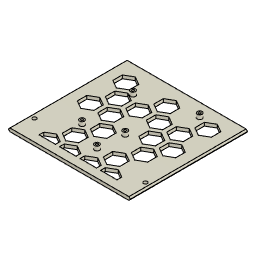
MCU Tray - BTT SKR E3 (Autodesk Fusion 360 design; units mm, degrees)
Autodesk Fusion 360 part; units mm, degrees
note: some values were not read from the file. Chosen so that the rebuilt part matches the saved one: a direction.
imported_body "Derived Base Feature3" makes body 1
imported_body "Derived Base Feature4" makes body 2
imported_body "Derived Base Feature5" makes body 3
imported_body "Derived Base Feature6" makes body 4
sketch "Base" plane through (0, 0, 0) normal (0, 1, 0) x (1, 0, 0)
  line L0 (72.5, 2) -> (-72.5, 2)
  line L1 (-72.5, 2) -> (-72.5, -2) construction
  line L2 (-72.5, -2) -> (72.5, -2)
  line L3 (72.5, -2) -> (72.5, 2) construction
  line L4 (72.5, 2) -> (-72.5, -2) construction
  line L5 (-72.5, 2) -> (72.5, -2) construction
  line L6 (-72.5, 0) -> (-74.3, 0) construction
  line L7 (-72.5, -2) -> (-74.3, -0.2)
  line L8 (-74.3, 0.2) -> (-72.5, 2)
  line L9 (-74.3, -0.2) -> (-74.3, 0)
  line L10 (-74.3, 0) -> (-74.3, 0.2)
  line L11 (0, 0) -> (0, -2) construction
  line L12 (72.5, -2) -> (74.3, -0.2)
  line L13 (74.3, -0.2) -> (74.3, 0)
  line L14 (74.3, 0) -> (74.3, 0.2)
  line L15 (74.3, 0.2) -> (72.5, 2)
  dimension "d1" = 145
  dimension "d2" = 4
  dimension "d3" = 0.2
  constraint horizontal L0
  constraint perpendicular L0 L1
  constraint parallel L0 L2
  constraint parallel L1 L3
  constraint coincident L4 L11.start
  constraint coincident L5 L11.start
  constraint coincident L11.start origin
  constraint midpoint L1 L6.start
  constraint perpendicular L1 L6
  constraint coincident L5 L0.end
  constraint coincident L0 L1.start
  constraint perpendicular L6 L9
  constraint perpendicular L6 L10
  constraint midpoint L2 L11.end
  constraint symmetric L1.end L11 L2.end
  constraint symmetric L0.end L11 L0.start
  constraint symmetric L7.end L11 L12.end
  constraint symmetric L6.end L11 L13.end
  constraint symmetric L8.start L11 L14.end
  measures "d1" distance of L1.end L2.end
  measures "d2" distance of L0.end L1.end
  measures "d3" distance of L7.end L6.end
extrude "Extrude1" add sketch "Base" along normal blind 190 and the other way blind 15 separate body makes body 5
sketch "Tray Mounting Holes" plane through (0, 0, 2) normal (0, 0, 1) x (-1, 0, 0)
  line L0 (72.5, 15) -> (-72.5, 15)
  line L1 (-72.5, 15) -> (-72.5, -190)
  line L2 (-72.5, -190) -> (72.5, -190)
  line L3 (72.5, -190) -> (72.5, 15)
  line L4 (0, 0) -> (0, -13.083) construction
  circle A0 centre (-67.6414, -16.9998) radius 2.3
  line L5 (72.6414, -59.8458) -> (72.6414, 0.0002) construction
  circle A1 centre (67.6414, -16.9998) radius 2.3
  line L6 (72.5, -190) -> (72.5, 15)
  line L7 (72.6414, 0.0002) -> (78.5, 0.0002)
  line L8 (72.6414, 0.0002) -> (67.6414, 0.0002) construction
  line L9 (67.6414, 0.0002) -> (67.6414, -16.9998) construction
  line L10 (67.6414, -16.9998) -> (72.6414, -16.9998) construction
  line L11 (72.6414, -16.9998) -> (72.6414, 0.0002) construction
  dimension "d14" = 5
  dimension "d15" = 17
  dimension "d16" = 4.6
  constraint coincident L4.start origin
  constraint vertical L4
  constraint symmetric L4 A0 A1
  constraint horizontal L8
  constraint vertical L9
  constraint horizontal L10
  constraint vertical L11
  constraint coincident L5.end L7.start
  constraint coincident A1.centre L9.end
  measures "d14" distance of L5.end L8.end
  measures "d15" distance of L5.end L10.end
  measures "d16" diameter of A1
extrude "Extrude2" cut sketch "Tray Mounting Holes" against normal up to surface (4 mm away) contours A0 | A1 bodies 5
extrude "Extrude3" cut 1 faces at (24.1667, 190, 0.6667) along direction (0, -1, 0) blind 40.154 on bodies 5 bodies 5
sketch "MCU Mount Standoffs" plane through (0, 0, 2) normal (0, 0, 1) x (-1, 0, 0)
  line L0 (-72.5, -149.846) -> (72.5, -149.846)
  line L1 (72.5, -149.846) -> (72.5, 15)
  line L2 (72.5, 15) -> (-72.5, 15)
  line L3 (-72.5, 15) -> (-72.5, -149.846)
  circle A0 centre (67.6414, -16.9998) radius 2.3
  circle A1 centre (-67.6414, -16.9998) radius 2.3
  circle A2 centre (-45, 10.1542) radius 3 construction
  circle A3 centre (-45, -139.8458) radius 3 construction
  line L4 (0, -126.2101) -> (0, -149.846) construction
  line L5 (0, -126.2101) -> (0, -22.8658) construction
  line L6 (-32.235, -22.8658) -> (32.235, -22.8658) construction
  line L7 (32.235, -22.8658) -> (32.235, -118.5458) construction
  line L8 (32.235, -118.5458) -> (-32.235, -118.5458) construction
  line L9 (-32.235, -118.5458) -> (-32.235, -22.8658) construction
  circle A4 centre (-32.235, -118.5458) radius 1.4
  circle A5 centre (-32.235, -118.5458) radius 3
  line L10 (32.235, -22.8658) -> (-2.745, -22.8658) construction
  circle A6 centre (-2.745, -22.8658) radius 1.4
  circle A7 centre (-2.745, -22.8658) radius 3
  line L11 (32.235, -22.8658) -> (-5.395, -22.8658) construction
  line L12 (-5.395, -22.8658) -> (-5.395, -54.6658) construction
  circle A8 centre (-5.395, -54.6658) radius 1.4
  circle A9 centre (-5.395, -54.6658) radius 3
  line L13 (32.235, -70.7058) -> (-32.235, -70.7058) construction
  circle A10 centre (32.235, -101.7808) radius 1.4
  circle A11 centre (32.235, -101.7808) radius 3
  circle A12 centre (32.235, -39.6308) radius 1.4
  circle A13 centre (32.235, -39.6308) radius 3
  point P0 (0, -75.2851)
  dimension "d60" = 64.47
  dimension "d61" = 95.68
  dimension "d62" = 2.8
  dimension "d63" = 6
  dimension "d64" = 34.98
  dimension "d65" = 2.8
  dimension "d66" = 6
  dimension "d67" = 37.63
  dimension "d68" = 31.8
  dimension "d69" = 2.8
  dimension "d70" = 6
  dimension "d73" = 2.8
  dimension "d74" = 6
  dimension "d75" = 62.15
  constraint midpoint L0 L4.end
  constraint vertical L4
  constraint vertical L5
  constraint horizontal L6
  constraint perpendicular L6 L7
  constraint parallel L6 L8
  constraint parallel L7 L9
  constraint coincident L8.end L9.start
  constraint coincident L6 L5.end
  constraint coincident L5 P0
  constraint perpendicular L7 L10
  constraint coincident L10.end A6.centre
  constraint perpendicular L7 L11
  constraint perpendicular L6 L12
  constraint coincident L12.end A8.centre
  constraint midpoint L7 L13.start
  constraint midpoint L9 L13.end
  constraint symmetric L13 A10 A12
  constraint symmetric L13 A11 A13
  constraint coincident L7 A10.centre
  constraint coincident A10.centre A11.centre
  measures "d60" distance of L7.end L8.end
  measures "d61" distance of L6.end L7.end
  measures "d62" diameter of A4
  measures "d63" diameter of A5
  measures "d64" distance of L6.end L10.end
  measures "d65" diameter of A6
  measures "d66" diameter of A7
  measures "d67" distance of L6.end L11.end
  measures "d68" distance of L11.end L12.end
  measures "d69" diameter of A8
  measures "d70" diameter of A9
  measures "d73" diameter of A10
  measures "d74" diameter of A11
  measures "d75" distance of A10.centre A12.centre
extrude "Extrude4" add sketch "MCU Mount Standoffs" along normal blind 5 contours A5 | A7 | A9 | A11 | A13 bodies 5
sketch "Vent Hexagons" plane through (0, 0, 2) normal (0, 0, 1) x (-1, 0, 0)
  line L0 (-72.5, -149.846) -> (72.5, -149.846)
  line L1 (72.5, -149.846) -> (72.5, 15)
  line L2 (72.5, 15) -> (-72.5, 15)
  line L3 (-72.5, 15) -> (-72.5, -149.846)
  circle A0 centre (67.6414, -16.9998) radius 2.3
  circle A1 centre (-67.6414, -16.9998) radius 2.3
  line L4 (0, -149.846) -> (0, 15) construction
  line L5 (72.5, -67.423) -> (-72.5, -67.423) construction
  line L6 (-10, -73.1965) -> (0, -78.97)
  line L7 (0, -78.97) -> (10, -73.1965)
  line L8 (10, -73.1965) -> (10, -61.6495)
  line L9 (10, -61.6495) -> (0, -55.876)
  line L10 (0, -55.876) -> (-10, -61.6495)
  line L11 (-10, -61.6495) -> (-10, -73.1965)
  line L12 (-25, -78.97) -> (-15, -73.1965)
  line L13 (-15, -73.1965) -> (-15, -61.6495)
  line L14 (-15, -61.6495) -> (-25, -55.876)
  line L15 (-25, -55.876) -> (-35, -61.6495)
  line L16 (-35, -61.6495) -> (-35, -73.1965)
  line L17 (-35, -73.1965) -> (-25, -78.97)
  line L18 (-12.5, -77.5266) -> (-22.5, -83.3001)
  line L19 (-22.5, -83.3001) -> (-22.5, -94.8471)
  line L20 (-22.5, -94.8471) -> (-12.5, -100.6206)
  line L21 (-12.5, -100.6206) -> (-2.5, -94.8471)
  line L22 (-2.5, -83.3001) -> (-12.5, -77.5266)
  line L23 (-2.5, -94.8471) -> (-2.5, -83.3001)
  line L24 (2.5, -83.3001) -> (2.5, -94.8471)
  line L25 (2.5, -94.8471) -> (12.5, -100.6206)
  line L26 (12.5, -100.6206) -> (22.5, -94.8471)
  line L27 (22.5, -94.8471) -> (22.5, -83.3001)
  line L28 (12.5, -77.5266) -> (2.5, -83.3001)
  line L29 (22.5, -83.3001) -> (12.5, -77.5266)
  line L30 (15, -73.1965) -> (25, -78.97)
  line L31 (25, -78.97) -> (35, -73.1965)
  line L32 (35, -73.1965) -> (35, -61.6495)
  line L33 (35, -61.6495) -> (25, -55.876)
  line L34 (15, -61.6495) -> (15, -73.1965)
  line L35 (25, -55.876) -> (15, -61.6495)
  line L36 (12.5, -57.3194) -> (22.5, -51.5459)
  line L37 (22.5, -51.5459) -> (22.5, -39.9989)
  line L38 (22.5, -39.9989) -> (12.5, -34.2254)
  line L39 (12.5, -34.2254) -> (2.5, -39.9989)
  line L40 (2.5, -51.5459) -> (12.5, -57.3194)
  line L41 (2.5, -39.9989) -> (2.5, -51.5459)
  line L42 (-2.5, -51.5459) -> (-2.5, -39.9989)
  line L43 (-2.5, -39.9989) -> (-12.5, -34.2254)
  line L44 (-12.5, -34.2254) -> (-22.5, -39.9989)
  line L45 (-22.5, -39.9989) -> (-22.5, -51.5459)
  line L46 (-12.5, -57.3194) -> (-2.5, -51.5459)
  line L47 (-22.5, -51.5459) -> (-12.5, -57.3194)
  line L48 (-60, -73.1965) -> (-50, -78.97)
  line L49 (-50, -78.97) -> (-40, -73.1965)
  line L50 (-40, -73.1965) -> (-40, -61.6495)
  line L51 (-40, -61.6495) -> (-50, -55.876)
  line L52 (-50, -55.876) -> (-60, -61.6495)
  line L53 (-60, -61.6495) -> (-60, -73.1965)
  line L54 (-50, -78.97) -> (-50, -67.423) construction
  line L55 (-50, -67.423) -> (-45, -76.0833) construction
  line L56 (-27.5, -94.8471) -> (-27.5, -83.3001)
  line L57 (-27.5, -83.3001) -> (-37.5, -77.5266)
  line L58 (-37.5, -77.5266) -> (-47.5, -83.3001)
  line L59 (-47.5, -83.3001) -> (-47.5, -94.8471)
  line L60 (-47.5, -94.8471) -> (-37.5, -100.6206)
  line L61 (-37.5, -100.6206) -> (-27.5, -94.8471)
  line L62 (-15, -116.4978) -> (-15, -104.9508)
  line L63 (-15, -104.9508) -> (-25, -99.1773)
  line L64 (-25, -99.1773) -> (-35, -104.9508)
  line L65 (-35, -104.9508) -> (-35, -116.4978)
  line L66 (-35, -116.4978) -> (-25, -122.2713)
  line L67 (-25, -122.2713) -> (-15, -116.4978)
  line L68 (-2.5, -138.1484) -> (-2.5, -126.6014)
  line L69 (-2.5, -126.6014) -> (-12.5, -120.8279)
  line L70 (-12.5, -120.8279) -> (-22.5, -126.6014)
  line L71 (-22.5, -126.6014) -> (-22.5, -138.1484)
  line L72 (-22.5, -138.1484) -> (-12.5, -143.9219)
  line L73 (-12.5, -143.9219) -> (-2.5, -138.1484)
  line L74 (-47.5, -51.5459) -> (-37.5, -57.3194)
  line L75 (-37.5, -57.3194) -> (-27.5, -51.5459)
  line L76 (-27.5, -51.5459) -> (-27.5, -39.9989)
  line L77 (-27.5, -39.9989) -> (-37.5, -34.2254)
  line L78 (-47.5, -39.9989) -> (-47.5, -51.5459)
  line L79 (-37.5, -34.2254) -> (-47.5, -39.9989)
  line L80 (-10, -116.4978) -> (0, -122.2713)
  line L81 (0, -122.2713) -> (10, -116.4978)
  line L82 (10, -116.4978) -> (10, -104.9508)
  line L83 (10, -104.9508) -> (0, -99.1773)
  line L84 (0, -99.1773) -> (-10, -104.9508)
  line L85 (-10, -104.9508) -> (-10, -116.4978)
  line L86 (2.5, -138.1484) -> (12.5, -143.9219)
  line L87 (12.5, -143.9219) -> (22.5, -138.1484)
  line L88 (22.5, -138.1484) -> (22.5, -126.6014)
  line L89 (22.5, -126.6014) -> (12.5, -120.8279)
  line L90 (2.5, -126.6014) -> (2.5, -138.1484)
  line L91 (12.5, -120.8279) -> (2.5, -126.6014)
  line L92 (2.5, -8.2446) -> (12.5, -14.0181)
  line L93 (12.5, -14.0181) -> (22.5, -8.2446)
  line L94 (22.5, -8.2446) -> (22.5, -2.4711)
  line L95 (2.5, -2.4711) -> (2.5, -8.2446)
  line L96 (-10, -29.8952) -> (0, -35.6687)
  line L97 (0, -35.6687) -> (10, -29.8952)
  line L98 (10, -29.8952) -> (10, -18.3482)
  line L99 (10, -18.3482) -> (0, -12.5747)
  line L100 (-10, -18.3482) -> (-10, -29.8952)
  line L101 (0, -12.5747) -> (-10, -18.3482)
  line L102 (-35, -29.8952) -> (-25, -35.6687)
  line L103 (-25, -35.6687) -> (-15, -29.8952)
  line L104 (-15, -29.8952) -> (-15, -18.3482)
  line L105 (-15, -18.3482) -> (-25, -12.5747)
  line L106 (-35, -18.3482) -> (-35, -29.8952)
  line L107 (-25, -12.5747) -> (-35, -18.3482)
  line L108 (27.5, -94.8471) -> (37.5, -100.6206)
  line L109 (37.5, -100.6206) -> (47.5, -94.8471)
  line L110 (47.5, -94.8471) -> (47.5, -83.3001)
  line L111 (47.5, -83.3001) -> (37.5, -77.5266)
  line L112 (27.5, -83.3001) -> (27.5, -94.8471)
  line L113 (37.5, -77.5266) -> (27.5, -83.3001)
  line L114 (40, -116.4978) -> (50, -122.2713)
  line L115 (50, -122.2713) -> (60, -116.4978)
  line L116 (60, -116.4978) -> (60, -104.9508)
  line L117 (60, -104.9508) -> (50, -99.1773)
  line L118 (40, -104.9508) -> (40, -116.4978)
  line L119 (50, -99.1773) -> (40, -104.9508)
  line L120 (15, -116.4978) -> (25, -122.2713)
  line L121 (25, -122.2713) -> (35, -116.4978)
  line L122 (35, -116.4978) -> (35, -104.9508)
  line L123 (35, -104.9508) -> (25, -99.1773)
  line L124 (15, -104.9508) -> (15, -116.4978)
  line L125 (25, -99.1773) -> (15, -104.9508)
  line L126 (0, -67.423) -> (35, -128.0448) construction
  line L127 (47.5, -51.5459) -> (37.5, -57.3194)
  line L128 (37.5, -57.3194) -> (27.5, -51.5459)
  line L129 (27.5, -51.5459) -> (27.5, -39.9989)
  line L130 (27.5, -39.9989) -> (37.5, -34.2254)
  line L131 (37.5, -34.2254) -> (47.5, -39.9989)
  line L132 (47.5, -39.9989) -> (47.5, -51.5459)
  line L133 (25, -35.6687) -> (15, -29.8952)
  line L134 (15, -29.8952) -> (15, -18.3482)
  line L135 (15, -18.3482) -> (25, -12.5747)
  line L136 (25, -12.5747) -> (35, -18.3482)
  line L137 (35, -29.8952) -> (25, -35.6687)
  line L138 (35, -18.3482) -> (35, -29.8952)
  line L139 (60, -73.1965) -> (50, -78.97)
  line L140 (50, -78.97) -> (40, -73.1965)
  line L141 (40, -73.1965) -> (40, -61.6495)
  line L142 (40, -61.6495) -> (50, -55.876)
  line L143 (60, -61.6495) -> (60, -73.1965)
  line L144 (50, -55.876) -> (60, -61.6495)
  line L145 (27.5, -2.4711) -> (27.5, -8.2446)
  line L146 (27.5, -8.2446) -> (37.5, -14.0181)
  line L147 (37.5, -14.0181) -> (47.5, -8.2446)
  line L148 (47.5, -8.2446) -> (47.5, -2.4711)
  line L149 (-60, -116.4978) -> (-50, -122.2713)
  line L150 (-50, -122.2713) -> (-40, -116.4978)
  line L151 (-40, -116.4978) -> (-40, -104.9508)
  line L152 (-40, -104.9508) -> (-50, -99.1773)
  line L153 (-50, -99.1773) -> (-60, -104.9508)
  line L154 (-60, -104.9508) -> (-60, -116.4978)
  line L155 (47.5, -2.4711) -> (27.5, -2.4711)
  line L156 (22.5, -2.4711) -> (2.5, -2.4711)
  line L157 (-2.5, -8.2446) -> (-2.5, -2.4711)
  line L158 (-2.5, -2.4711) -> (-22.5, -2.4711)
  line L159 (-22.5, -2.4711) -> (-22.5, -8.2446)
  line L160 (-22.5, -8.2446) -> (-12.5, -14.0181)
  line L161 (-12.5, -14.0181) -> (-2.5, -8.2446)
  line L162 (-27.5, -2.4711) -> (-47.5, -2.4711)
  line L163 (-47.5, -2.4711) -> (-47.5, -8.2446)
  line L164 (-47.5, -8.2446) -> (-37.5, -14.0181)
  line L165 (-27.5, -8.2446) -> (-27.5, -2.4711)
  line L166 (-37.5, -14.0181) -> (-27.5, -8.2446)
  circle A2 centre (-2.745, -22.8658) radius 3
  circle A3 centre (-5.395, -54.6658) radius 3
  circle A4 centre (32.235, -39.6308) radius 3
  circle A5 centre (32.235, -101.7808) radius 3
  circle A6 centre (-32.235, -118.5458) radius 3
  point P0 (0, -67.423)
  dimension "d27" = 10
  dimension "d29" = 360
  dimension "d32" = 25
  dimension "d33" = 0
  constraint midpoint L0 L4.start
  constraint midpoint L2 L4.end
  constraint midpoint L1 L5.start
  constraint midpoint L3 L5.end
  constraint midpoint L5 P0
  constraint coincident L5 L54.end
  constraint perpendicular L5 L54
  constraint midpoint L49 L55.end
  constraint perpendicular L49 L55
  constraint coincident P0 L126.start
  constraint perpendicular L115 L126
  constraint parallel L55 L126
  constraint symmetric L51.end L126 L134.end
  constraint symmetric L52.end L126 L135.end
  constraint symmetric L48.end L126 L137.start
  constraint symmetric L48.start L126 L136.end
  constraint symmetric L49.end L126 L133.start
  constraint symmetric L50.end L126 L133.end
  constraint symmetric L56.start L126 L127.end
  constraint symmetric L56.end L126 L128.end
  constraint symmetric L57.end L126 L129.end
  constraint symmetric L58.end L126 L130.end
  constraint symmetric L59.end L126 L131.end
  constraint symmetric L60.end L126 L127.start
  constraint symmetric L62.start L126 L139.end
  constraint symmetric L62.end L126 L140.end
  constraint symmetric L63.end L126 L141.end
  constraint symmetric L64.end L126 L142.end
  constraint symmetric L65.end L126 L143.start
  constraint symmetric L66.end L126 L139.start
  constraint collinear L155 L156
  constraint collinear L158 L162
  measures "d27" distance of P0 L11
extrude "Extrude5" cut sketch "Vent Hexagons" against normal blind 4 contours L12 L13 L14 L15 L16 L17 | L18 L19 L20 L21 L22 L23 | L24 L25 L26 L27 L28 L29 | L30 L31 L32 L33 L34 L35 | L36 L37 L38 L39 L40 L41 | L48 L49 L50 L51 L52 L53 | L56 L57 L58 L59 L60 L61 | L74 L75 L76 L77 L78 L79 | L80 L81 L82 L83 L84 L85 | L92 L93 L94 L95 L156 | L102 L103 L104 L105 L106 L107 | L108 L109 L110 L111 L112 L113 | L114 L115 L116 L117 L118 L119 | L133 L134 L135 L136 L137 L138 | L139 L140 L141 L142 L143 L144 | L145 L146 L147 L148 L155 | L149 L150 L151 L152 L153 L154 | L157 L158 L159 L160 L161 | L162 L163 L164 L165 L166 bodies 5
extrude "Extrude6" cut 1 faces at (24.1667, -15, 0.6667) along direction (0, 1, 0) blind 7 on bodies 5 bodies 5
extrude "Extrude7" cut 1 faces at (24.1667, 149.846, 0.6667) along direction (0, -1, 0) blind 15 on bodies 5 bodies 5
hidden bodies 1 2 3 4
named bodies: "Body1 (Context4)", "Body1 (1) (Context4)", "Body1 (2) (Context4)", "Body1 (3) (Context4)"
